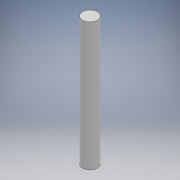
# Autodesk Inventor part: Stav
Saved by Autodesk Inventor 2018 (Build 220112000, 112)
## iProperties
Created: 2018-02-08
Part Number: Stav
Material: Generic
Document SubType Name: Modeling
Designer: davton
Density: 1 g/cm^3
Appearance: Default
Author: davton
Autodesk Inventor part; units mm, degrees
ref_plane "YZ Plane" through (0, 0, 0) normal (1, 0, 0) x (0, 1, 0)
ref_plane "XZ Plane" through (0, 0, 0) normal (0, 1, 0) x (-1, 0, 0)
ref_plane "XY Plane" through (0, 0, 0) normal (0, 0, 1) x (1, 0, 0)
sketch "Sketch1" plane through (0, 0, 0) normal (0, 0, 1) x (1, 0, 0)
  circle A0 centre (0, 0) radius 1.3333
  dimension "d1" = 2.6667
  constraints: 1 centre point, 1 coincident
  measures "d1" diameter of A0
extrude "Extrusion1" add sketch "Sketch1" along normal blind 23.3333
sketch "Sketch2" plane through (0, 0, 0) normal (0, 1, 0) x (-1, 0, 0)
  point P0 (0, 0)
equation "\"d1\" = 0.666667 * HD"
equation "\"d2\" = 0.56 * HL"
equation "\"HD\" = 4"
equation "\"HL\" = 41.66667"
body "Solid1"
